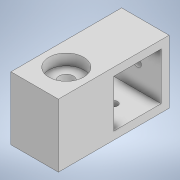
# Autodesk Inventor part: double_gear_mount
Saved by Autodesk Inventor 2022.3 (Build 263350000, 350)
## iProperties
Created: 2022-06-10
Part Number: double_gear_mount
Material: Generic
Document SubType Name: Modeling
Designer: Martijn
Density: 1 g/cm^3
Appearance: Default
Author: Martijn
Autodesk Inventor part; units mm, degrees
ref_plane "YZ Plane" through (0, 0, 0) normal (1, 0, 0) x (0, 1, 0)
ref_plane "XZ Plane" through (0, 0, 0) normal (0, 1, 0) x (-1, 0, 0)
ref_plane "XY Plane" through (0, 0, 0) normal (0, 0, 1) x (1, 0, 0)
sketch "Sketch1" plane through (0, 0, 0) normal (0, 0, 1) x (1, 0, 0)
  line L0 (0, 0) -> (30, 0)
  line L1 (30, 0) -> (30, 40)
  line L2 (30, 40) -> (0, 40)
  line L3 (0, 40) -> (0, 0)
  dimension "d0" = 40
  dimension "d1" = 30
  constraints: 8 end point, 2 parallel, 1 horizontal, 1 perpendicular
  measures "d0" distance of L0.end L1.end
  measures "d1" distance of L0.start L0.end
extrude "Extrusion1" add sketch "Sketch1" along normal blind 70
sketch "Sketch2" plane through (30, 0, 0) normal (1, 0, 0) x (0, 0, -1)
  line L0 (-5, 5) -> (-35, 5)
  line L1 (-35, 5) -> (-35, 35)
  line L2 (-35, 35) -> (-5, 35)
  line L3 (-5, 35) -> (-5, 5)
  line L4 (0, 0) -> (0, 40) projected
  line L5 (0, 0) -> (-70, 0) projected
  point P0 (-5, 20)
  dimension "d4" = 5
  dimension "d5" = 30
  dimension "d6" = 30
  dimension "d7" = 5
  constraints: 8 end point, 2 parallel, 1 horizontal, 1 midpoint, 1 perpendicular
  measures "d4" distance between parallel lines of L4 L3
  measures "d5" distance from line of point (-5, 20) L1
  measures "d6" distance between parallel lines of L0 L2
  measures "d7" distance between parallel lines of L5 L0
extrude "Extrusion2" cut sketch "Sketch2" against normal blind 70
sketch "Sketch3" plane through (0, 0, 0) normal (0, -1, 0) x (1, 0, 0)
  circle A0 centre (15, 50) radius 11
  line L0 (30, 35) -> (0, 35) projected
  line L1 (30, 0) -> (30, 70) projected
  point P0 (0, 0)
  dimension "d10" = 15
  dimension "d11" = 22
  dimension "d12" = 15
  constraints: 1 centre point
  measures "d10" distance from line of L0 A0.centre
  measures "d11" diameter of A0
  measures "d12" distance from line of L1 A0.centre
extrude "Extrusion3" cut sketch "Sketch3" against normal blind 7
sketch "Sketch4" plane through (0, 40, 0) normal (0, 1, 0) x (1, 0, 0)
  circle A0 centre (15, -50) radius 11
  line L0 (0, 0) -> (0, -70) projected
  point P0 (30, -35)
  dimension "d15" = 22
  dimension "d16" = 15
  dimension "d17" = 15
  constraints: 1 centre point
  measures "d15" diameter of A0
  measures "d16" distance from line of L0 A0.centre
  measures "d17" horizontal distance of A0.centre point (30, -35)
extrude "Extrusion4" cut sketch "Sketch4" against normal blind 7
sketch "Sketch5" plane through (15, 33, 50) normal (0, 1, 0) x (1, 0, 0)
  circle A0 centre (0, 0) radius 4.5
  point P0 (-15, 50)
  dimension "d20" = 9
  constraints: 1 centre point
  measures "d20" diameter of A0
extrude "Extrusion5" cut sketch "Sketch5" against normal blind 30
sketch "Sketch6" plane through (0, 0, 0) normal (0, -1, 0) x (1, 0, 0)
  circle A0 centre (15, 20) radius 2.5
  line L0 (0, 0) -> (0, 70) projected
  point P0 (0, 5)
  dimension "d23" = 5
  dimension "d24" = 15
  dimension "d25" = 15
  constraints: 1 centre point
  measures "d23" diameter of A0
  measures "d24" distance from line of L0 A0.centre
  measures "d25" horizontal distance of point (0, 5) A0.centre
extrude "Extrusion6" cut sketch "Sketch6" against normal blind 10
sketch "Sketch7" plane through (0, 0, 0) normal (0, 0, -1) x (-1, 0, 0)
  circle A0 centre (-15, 20) radius 2.5
  line L0 (0, 40) -> (0, 0) projected
  point P0 (0, 5)
  dimension "d28" = 5
  dimension "d29" = 15
  dimension "d30" = 15
  constraints: 1 centre point
  measures "d28" diameter of A0
  measures "d29" distance from line of A0.centre L0
  measures "d30" horizontal distance of point (0, 5) A0.centre
extrude "Extrusion7" cut sketch "Sketch7" against normal blind 10
body "Solid1"
